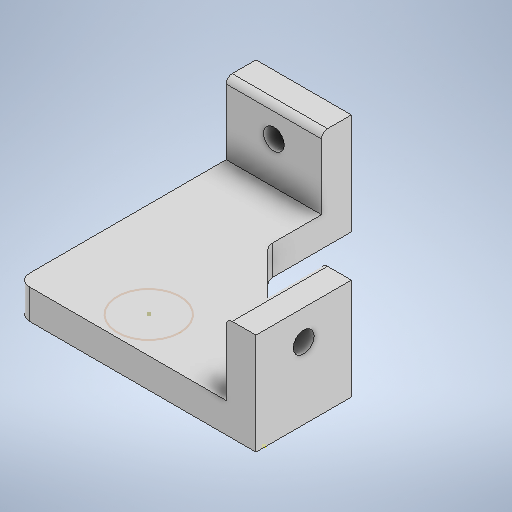
# Autodesk Inventor part: C4-T-B-case-bracket
Saved by Autodesk Inventor 2025.2 (Build 292293000, 293)
## iProperties
Created: 2025-11-15
Part Number: C4-T-B-case-bracket
Material: 일반
Document SubType Name: Modeling
Designer: RunGeun
Density: 1 g/cm^3
Appearance: 기본값
Author: RunGeun
Autodesk Inventor part; units mm, degrees
ref_plane "YZ Plane" through (0, 0, 0) normal (1, 0, 0) x (0, 1, 0)
ref_plane "XZ Plane" through (0, 0, 0) normal (0, 1, 0) x (-1, 0, 0)
ref_plane "XY Plane" through (0, 0, 0) normal (0, 0, 1) x (1, 0, 0)
sketch "스케치1" plane through (0, 0, 0) normal (0, 1, 0) x (-1, 0, 0)
  line L0 (39.7893, 1.5034) -> (-0.2107, 1.5034)
  line L1 (-0.2107, 1.5034) -> (-0.2107, -14.4966)
  line L2 (23.7893, -38.4966) -> (39.7893, -38.4966)
  line L3 (39.7893, -38.4966) -> (39.7893, 1.5034)
  line L4 (23.7893, -14.4966) -> (-0.2107, -14.4966)
  line L5 (23.7893, -38.4966) -> (23.7893, -14.4966)
  line L6 (23.7893, -38.4966) -> (39.7893, -38.4966)
  line L7 (39.7893, -38.4966) -> (39.7893, -33.4966)
  line L8 (39.7893, -33.4966) -> (23.7893, -33.4966)
  line L9 (23.7893, -33.4966) -> (23.7893, -38.4966)
  line L10 (-0.2107, -14.4966) -> (4.7893, -14.4966)
  line L11 (4.7893, -14.4966) -> (4.7893, 1.5034)
  line L12 (4.7893, 1.5034) -> (-0.2107, 1.5034)
  line L13 (-0.2107, 1.5034) -> (-0.2107, -14.4966)
  point P0 (0, 0)
  point P1 (4.7893, -14.4966)
  point P2 (23.7893, -33.4966)
  dimension "d10" = 5
  dimension "d11" = 5
  dimension "d31" = 16
  dimension "d32" = 16
  dimension "d38" = 40
  dimension "d39" = 40
  constraints: 28 end point, 6 parallel, 4 horizontal, 3 perpendicular, 2 point on line
  measures "d10" distance of L7.end L6.end
  measures "d11" distance of L12.end L11.end
  measures "d31" distance of L0.end L1.end
  measures "d32" distance of L2.start L2.end
  measures "d38" distance of L2.end L0.start
  measures "d39" distance of L0.start L0.end
extrude "돌출1" add sketch "스케치1" along normal blind 5 contours L3 L8 L5 L4 L11 L0
extrude "돌출2" add sketch "스케치1" along normal blind 17 contours L11 L4 L1 L0 | L3 L2 L5 L8
chamfer "모따기1" distance 10 angle 45 1 edges at (-23.7893, 2.5, -14.4966)
fillet "모깎기1" radius 2 3 edges at (-39.7893, 2.5, 1.5034) (-13.7893, 2.5, -14.4966) (-23.7893, 2.5, -24.4966)
sketch "스케치2" plane through (-4.7893, 5, 1.5034) normal (-1, 0, 0) x (0, 0, 1)
  circle A0 centre (-8, 7) radius 1.75
  line L0 (0, 0) -> (0, 12) projected
  line L1 (-16, 12) -> (0, 12) projected
  point P0 (-1.5034, -5)
  dimension "d20" = 3.5
  dimension "d21" = 8
  dimension "d22" = 5
  constraints: 1 centre point
  measures "d20" diameter of A0
  measures "d21" distance from line of L0 A0.centre
  measures "d22" distance from line of A0.centre L1
extrude "돌출3" cut sketch "스케치2" against normal blind 20
sketch "스케치3" plane through (-39.7893, 5, -33.4966) normal (0, 0, 1) x (1, 0, 0)
  circle A0 centre (8, 7) radius 1.75
  line L0 (16, 0) -> (16, 12) projected
  line L1 (0, 12) -> (16, 12) projected
  point P0 (39.7893, -5)
  dimension "d25" = 3.5
  dimension "d26" = 8
  dimension "d27" = 5
  constraints: 1 centre point
  measures "d25" diameter of A0
  measures "d26" distance from line of A0.centre L0
  measures "d27" distance from line of A0.centre L1
extrude "돌출4" cut sketch "스케치3" against normal blind 20
fillet "모깎기2" radius 1 2 edges at (-31.7893, 17, -33.4966) (-4.7893, 17, -6.4966)
sketch "스케치4" plane through (0, 0, 0) normal (0, -1, 0) x (1, 0, 0)
  circle A0 centre (-28.7893, -9.4966) radius 5.25
  line L0 (-39.7893, -38.4966) -> (-39.7893, -0.4966) projected
  line L1 (-37.7893, 1.5034) -> (0.2107, 1.5034) projected
  point P0 (0, 0)
  dimension "d33" = 10.5
  dimension "d34" = 11
  dimension "d35" = 11
  constraints: 1 centre point
  measures "d33" diameter of A0
  measures "d34" distance from line of L0 A0.centre
  measures "d35" distance from line of L1 A0.centre
extrude "돌출5" cut sketch "스케치4" against normal blind 0.8
sketch "스케치5" plane through (0, 0, 0) normal (0, -1, 0) x (1, 0, 0)
  circle A0 centre (-28.7893, -9.4966) radius 5.25 projected
  circle A1 centre (-28.7893, -9.4966) radius 5.25
  point P0 (0, 0)
  constraints: 1 centre point, 1 coincident
equation "\"d39\" = d38"
equation "\"d35\" = d34"
